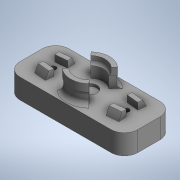
# Autodesk Inventor part: MG996R Arm Test
Saved by Autodesk Inventor 2020.5 (Build 245400000, 400)
## iProperties
Created: 2023-03-16
Part Number: MG996R Arm Test
Material: Generic
Document SubType Name: Modeling
Designer: Wes
Density: 1 g/cm^3
Appearance: Default
Author: Wes
Autodesk Inventor part; units mm, degrees
ref_plane "YZ Plane" through (0, 0, 0) normal (1, 0, 0) x (0, 1, 0)
ref_plane "XZ Plane" through (0, 0, 0) normal (0, 1, 0) x (-1, 0, 0)
ref_plane "XY Plane" through (0, 0, 0) normal (0, 0, 1) x (1, 0, 0)
sketch "Base" plane through (0, 0, 0) normal (0, 0, 1) x (1, 0, 0)
  line L0 (0, 0) -> (-22, 0)
  line L1 (-22, 0) -> (-22, 53)
  line L2 (-22, 53) -> (0, 53)
  line L3 (0, 53) -> (0, 0)
  line L4 (-11, 26.5) -> (-11, 43.6) construction
  line L5 (-11, 26.5) -> (-11, 9.4) construction
  line L6 (-11, 26.5) -> (-11, 10.7) construction
  line L7 (-11, 26.5) -> (-11, 42.3) construction
  line L8 (-11, 10.7) -> (-11, 9.4) construction
  line L9 (-11, 42.3) -> (-11, 43.6) construction
  circle A0 centre (-11, 42.95) radius 1.175
  circle A1 centre (-11, 10.05) radius 1.175
  dimension "d0" = 22
  dimension "d1" = 53
  dimension "d8" = 34.2
  dimension "d14" = 31.6
  dimension "d15" = 2.35
  dimension "d16" = 2.35
  constraints: 20 end point, 3 vertical, 2 centre point, 2 midpoint, 2 parallel, 2 point on line, 1 coincident, 1 collinear, 1 horizontal, 1 perpendicular
  measures "d0" distance of L1.end L2.end
  measures "d1" distance of L0.end L1.end
  measures "d8" distance of L4.end L5.end
  measures "d14" distance of L7.end L6.end
  measures "d15" diameter of A0
  measures "d16" diameter of A1
extrude "Extrusion1" add sketch "Base" along normal mid plane 9
sketch "Countersink Arm Screw Holes" plane through (0, 0, -4.5) normal (0, 0, -1) x (-1, 0, 0)
  circle A0 centre (11, 10.05) radius 1.175 projected
  circle A1 centre (11, 10.05) radius 2.7
  circle A2 centre (11, 42.95) radius 1.175 projected
  circle A3 centre (11, 42.95) radius 2.7
  point P0 (0, 0)
  dimension "d19" = 5.4
  dimension "d20" = 5.4
  constraints: 2 centre point, 2 coincident
  measures "d19" diameter of A1
  measures "d20" diameter of A3
extrude "Extrusion2" cut sketch "Countersink Arm Screw Holes" against normal blind 1.5 contours A0 | A1 | A2 | A3
sketch "Axle Screw Countersink" plane through (0, 0, 4.5) normal (0, 0, 1) x (1, 0, 0)
  circle A0 centre (-11, 26.5) radius 3.15
  point P0 (0, 0)
  dimension "d66" = 6.3
  constraints: 1 centre point, 1 coincident
  measures "d66" diameter of A0
extrude "Extrusion3" cut sketch "Axle Screw Countersink" against normal blind 1.2
sketch "Arm Center Fitting" plane through (0, 0, 4.5) normal (0, 0, 1) x (1, 0, 0)
  circle A0 centre (-11, 26.5) radius 5.975 construction
  line L0 (-6.6169, 22.4393) -> (-6.5972, 30.5393) construction
  line L1 (-6.6169, 22.4393) -> (-15.4028, 22.4607) construction
  line L2 (-15.4028, 22.4607) -> (-15.3831, 30.5607) construction
  arc A1 (-15.3831, 30.5607) -> (-15.4028, 22.4607) centre (-11, 26.5) ccw
  line L3 (-15.4028, 22.4607) -> (-17.245, 20.7706)
  line L4 (-15.3831, 30.5607) -> (-17.217, 32.2597)
  arc A2 (-17.217, 32.2597) -> (-17.245, 20.7706) centre (-11, 26.5) ccw
  line L5 (-11, 15.8409) -> (-11, 38.1893) construction
  arc A3 (-6.6169, 22.4393) -> (-6.5972, 30.5393) centre (-11, 26.5) ccw
  line L6 (-6.6169, 22.4393) -> (-4.755, 20.7706)
  line L7 (-6.5972, 30.5393) -> (-4.783, 32.2597)
  arc A4 (-4.755, 20.7706) -> (-4.783, 32.2597) centre (-11, 26.5) ccw
  point P0 (0, 0)
  dimension "d27" = 11.95
  dimension "d31" = 8.1
  dimension "d32" = 8.1
  dimension "d33" = 2.5
  dimension "d34" = 2.5
  constraints: 16 end point, 12 point on circle, 5 centre point, 2 line through centre, 2 symmetric about line, 1 concentric, 1 perpendicular, 1 vertical, 2 other
  measures "d27" diameter of A0
  measures "d31" distance of L0.start L0.end
  measures "d32" distance of L1.end L2.end
  measures "d33" distance of L1.end L3.end
  measures "d34" distance of L2.end L4.end
extrude "Extrusion4" add sketch "Arm Center Fitting" along normal blind 5
sketch "Rotation Support" plane through (0, 0, 9.5) normal (0, 0, 1) x (1, 0, 0)
  line L0 (-16.975, 26.5) -> (-17.775, 26.5) construction
  circle A0 centre (-11, 26.5) radius 6.775 construction
  arc A1 (-15.9844, 31.0887) -> (-15.9778, 21.9042) centre (-11, 26.5) ccw
  line L1 (-17.775, 26.5) -> (-19.775, 26.5) construction
  circle A2 centre (-11, 26.5) radius 8.775 construction
  arc A3 (-17.4516, 32.4479) -> (-17.4516, 20.5521) centre (-11, 26.5) ccw
  line L2 (-17.4516, 20.5521) -> (-15.9778, 21.9042)
  line L3 (-15.4028, 22.4607) -> (-17.245, 20.7706) projected
  line L4 (-15.9844, 31.0887) -> (-17.4516, 32.4479)
  line L5 (-17.217, 32.2597) -> (-15.3831, 30.5607) projected
  line L6 (-11, 15.0295) -> (-11, 38.5479) construction
  arc A4 (-6.0222, 21.9042) -> (-6.0156, 31.0887) centre (-11, 26.5) ccw
  arc A5 (-4.5484, 20.5521) -> (-4.5484, 32.4479) centre (-11, 26.5) ccw
  line L7 (-4.5484, 20.5521) -> (-6.0222, 21.9042)
  line L8 (-6.0156, 31.0887) -> (-4.5484, 32.4479)
  point P0 (0, 0)
  dimension "d38" = 0.8
  dimension "d39" = 2
  constraints: 16 point on circle, 10 end point, 6 centre point, 4 symmetric about line, 2 coincident, 2 horizontal, 1 concentric, 1 vertical, 10 other
  measures "d38" distance of L0.start L0.end
  measures "d39" distance of L0.end L1.end
extrude "Extrusion5" add sketch "Rotation Support" along normal blind 3.35
sketch "Arm Support" plane through (0, 0, 4.5) normal (0, 0, 1) x (1, 0, 0)
  circle A0 centre (-11, 10.05) radius 1.175 construction
  line L0 (-11, 8.875) -> (-11, 13.375) construction
  line L1 (-11, 13.375) -> (-7.875, 13.375) construction
  line L2 (-11, 13.375) -> (-14.125, 13.375) construction
  line L3 (-17.0644, 26.7154) -> (-5.1144, 26.7154) construction
  line L4 (-11, 10.05) -> (-8.2, 10.05) construction
  line L5 (-11, 10.05) -> (-8.2, 10.05) construction
  line L6 (-11, 10.05) -> (-13.8, 10.05) construction
  line L7 (-11, 10.05) -> (-8.2, 10.05) construction
  line L8 (-14.125, 13.375) -> (-13.8, 10.05)
  line L9 (-13.8, 10.05) -> (-15.7905, 9.8554)
  line L10 (-15.7905, 9.8554) -> (-16.1155, 13.1804)
  line L11 (-16.1155, 13.1804) -> (-14.125, 13.375)
  line L12 (-7.875, 13.375) -> (-8.2, 10.05)
  line L13 (-8.2, 10.05) -> (-6.2095, 9.8554)
  line L14 (-6.2095, 9.8554) -> (-5.8845, 13.1804)
  line L15 (-5.8845, 13.1804) -> (-7.875, 13.375)
  line L16 (-13.8, 10.05) -> (-13.6054, 8.0595)
  line L17 (-13.6054, 8.0595) -> (-15.596, 7.8649)
  line L18 (-15.596, 7.8649) -> (-15.7905, 9.8554)
  line L19 (-8.2, 10.05) -> (-8.3946, 8.0595)
  line L20 (-8.3946, 8.0595) -> (-6.404, 7.8649)
  line L21 (-6.404, 7.8649) -> (-6.2095, 9.8554)
  line L22 (-14.125, 40.0559) -> (-13.8, 43.3809)
  line L23 (-13.8, 43.3809) -> (-15.7905, 43.5755)
  line L24 (-15.7905, 43.5755) -> (-16.1155, 40.2505)
  line L25 (-16.1155, 40.2505) -> (-14.125, 40.0559)
  line L26 (-7.875, 40.0559) -> (-8.2, 43.3809)
  line L27 (-8.2, 43.3809) -> (-6.2095, 43.5755)
  line L28 (-5.8845, 40.2505) -> (-7.875, 40.0559)
  line L29 (-6.2095, 43.5755) -> (-5.8845, 40.2505)
  line L30 (-13.8, 43.3809) -> (-13.6054, 45.3714)
  line L31 (-13.6054, 45.3714) -> (-15.596, 45.566)
  line L32 (-15.596, 45.566) -> (-15.7905, 43.5755)
  line L33 (-8.2, 43.3809) -> (-8.3946, 45.3714)
  line L34 (-8.3946, 45.3714) -> (-6.404, 45.566)
  line L35 (-6.404, 45.566) -> (-6.2095, 43.5755)
  point P0 (0, 0)
  dimension "d45" = 4.5
  dimension "d51" = 6.25
  dimension "d63" = 5.6
  dimension "d64" = 2
  dimension "d65" = 2
  constraints: 72 end point, 18 symmetric about line, 7 horizontal, 5 perpendicular, 2 collinear, 1 vertical, 1 vertical alignment, 1 other
  measures "d45" distance of L0.start L0.end
  measures "d51" distance of L2.end L1.end
  measures "d63" distance of L6.end L4.end
  measures "d64" distance of L6.end L9.end
  measures "d65" distance of L6.end L16.end
extrude "Extrusion6" add sketch "Arm Support" along normal blind 3
draft "FaceDraft1" angle 28 pull direction (0, 0, 1) faces at (-6.2309, 9.6368, 5.5) (-6.0577, 42.0223, 5.5) fixed edges at (-6.1443, 10.5227, 7.5) (-6.1443, 42.9082, 7.5)
draft "FaceDraft2" angle 28 pull direction (0, 0, 1) faces at (-15.9423, 11.4086, 5.5) (-15.7691, 43.7941, 5.5) fixed edges at (-15.8557, 10.5227, 7.5) (-15.8557, 42.9082, 7.5)
fillet "Fillet1" radius 2 6 edges at (-17.775, 26.5058, 9.5) (-4.225, 26.4959, 9.5) (-19.475, 26.5206, 4.5) (-2.525, 26.5206, 4.5) (-19.475, 26.5099, 9.5) (-2.525, 26.5099, 9.5)
fillet "Fillet2" radius 6 4 edges at (0, 0, 0) (0, 53, 0) (-22, 53, 0) (-22, 0, 0)
body "Solid1"
